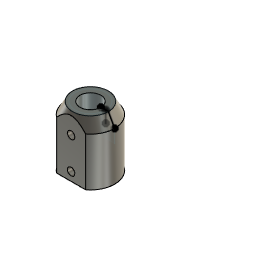
PuffingNozzle (Autodesk Fusion 360 design; units mm, degrees)
Autodesk Fusion 360 part; units mm, degrees
sketch "Sketch1" plane through (0, 0, 0) normal (0, 1, 0) x (1, 0, 0)
sketch "Sketch2" plane through (0, 0, 0) normal (0, 0, 1) x (1, 0, 0)
  circle A0 centre (-17.8237, 9.2304) radius 2.7432
  circle A1 centre (-17.8237, 9.2304) radius 6.35
  line L0 (-21.6337, 4.1504) -> (-14.0137, 4.1504)
  dimension "d3" = 5.4864
  dimension "d4" = 12.7
  dimension "d5" = 5.08
  constraint concentric A0 A1
  constraint coincident A1 L0.start
  constraint coincident A1 L0.end
  constraint horizontal L0
  measures "d3" diameter of A0
  measures "d4" diameter of A1
  measures "d5" distance of A0.centre L0
ref_plane "WorkPlane1" through (-17.8237, 9.2304, 2.9972) normal (0, 0, 1) x (1, 0, 0)
sketch "Sketch3" plane through (-17.8237, 9.2304, 2.9972) normal (0, 0, 1) x (1, 0, 0)
  circle A0 centre (0, 0) radius 4.0161
  constraint coincident A0.centre origin
extrude "Extrude1" add sketch "Sketch3" against normal up to surface (2.9972 mm away) makes body 1
extrude "Extrude2" cut sketch "Sketch2" along normal up to surface (2.9972 mm away) contours A0 bodies 1
extrude "Extrude3" add sketch "Sketch2" against normal blind 3.4544 bodies 1
sketch "Sketch4" plane through (0, 0, 0) normal (1, 0, 0) x (0, 1, 0)
ref_plane "WorkPlane2" through (0, 9.2202, 0) normal (0, 1, 0) x (0, 0, 1)
extrude "Extrude4" cut sketch "Sketch2" against normal blind 0.889 contours A1 L0 picked at (-18.8394, 3.9867) bodies 1
ref_plane "WorkPlane3" through (-17.8237, 9.2304, -0.4445) normal (0, -1, 0) x (-1, 0, 0)
extrude "Extrude5" add 1 faces at (-18.8394, 3.9867, -0.889) along direction (0, 0, 1) up to surface (0.889 mm away) on bodies 1 bodies 1
sketch "Sketch5" plane through (-17.8237, 9.2304, -0.4445) normal (0, -1, 0) x (1, 0, 0)
split "Split1" by plane through (-17.8237, 9.2304, -0.4445) normal (0, -1, 0) bodies 1 makes body 2 at (-11.5053, 8.5982, -2.3029)
sketch "Sketch6" plane through (-17.8237, 9.2304, -0.4445) normal (0, -1, 0) x (1, 0, 0)
sketch "Sketch7" plane through (0, 9.2304, 0) normal (0, -1, 0) x (1, 0, 0)
  line L0 (-11.4737, -3.4544) -> (-11.4737, 0)
  line L1 (-11.4737, 0) -> (-13.8076, 0)
  line L2 (-13.8076, 0) -> (-13.8076, 2.9972)
  line L3 (-13.8076, 2.9972) -> (-15.0805, 2.9972)
  line L4 (-15.0805, 2.9972) -> (-15.0805, -3.4544)
  line L5 (-15.0805, -3.4544) -> (-11.4737, -3.4544)
  line L6 (-13.8076, 0) -> (-13.8076, 2.9972)
  line L7 (-15.0805, 2.9972) -> (-13.1247, 2.9972)
  line L8 (-13.1247, 2.9972) -> (-11.4737, 0)
  dimension "d38" = 2.9972
  dimension "d39" = 1.9558
  constraint coincident L1.end L2.start
  constraint perpendicular L1 L6
  constraint coincident L3.end L4.start
  constraint perpendicular L2 L7
  constraint coincident L0.end L1.start
  measures "d38" distance of L1.end L2.end
  measures "d39" distance of L3.end L7.end
revolve "Revolve1" add sketch "Sketch7" angle 360 about axis through (-17.8237, 9.2304, 4.4958) along (0, 0, -1) contours L0 L1 L2 L3 L4 L5 L6 L7 bodies 1 2
extrude "Extrude6" cut sketch "Sketch2" against normal blind 6.35 contours A1 L0 picked at (-18.8394, 3.9867) bodies 1
extrude "Extrude7" add sketch "Sketch2" along normal blind 2.8194 separate body contours A1 L0 picked at (-18.8394, 3.9867) makes body 3
extrude "Extrude8" cut 1 faces at (-18.8394, 3.9867, 2.8194) along direction (0, 0, -1) blind 6.9088 on bodies 3 bodies 1 3
extrude "Extrude9" cut 1 faces at (-17.7554, 4.9319, -3.4544) along direction (0, 0, 1) blind 3.4544 on bodies 1 bodies 1
extrude "Extrude10" add sketch "Sketch2" against normal blind 18.6182 contours A1 L0 picked at (-17.7554, 4.9319) bodies 1 3
sketch "Sketch8" plane through (0, 4.1504, 0) normal (0, -1, 0) x (1, 0, 0)
  circle A0 centre (-17.8237, -10.4648) radius 0.9779
  circle A1 centre (-17.8237, -2.159) radius 0.9779
  line L0 (-14.0137, 0) -> (-21.6337, 0)
  dimension "d30" = 1.9558
  dimension "d32" = 1.9558
  dimension "d44" = 2.159
  dimension "d51" = 8.3058
  measures "d30" diameter of A0
  measures "d32" diameter of A1
  measures "d44" distance of A1.centre L0
  measures "d51" distance of A0.centre A1.centre
extrude "Extrude11" cut 1 faces at (-17.892, 4.9319, -18.6182) along direction (0, 0, 1) blind 1.6256 on bodies 1 bodies 1
surface "Revolve2" add revolved angle 360 about axis through (-17.8237, 9.2304, 4.4958) along (0, 0, -5.9944) profiles "Sketch7" section 1 contours L1 L2 L6 L7 L8 separate body makes body 4
sketch "Sketch9" plane through (0, 4.1504, 0) normal (0, -1, 0) x (1, 0, 0)
  line L0 (-21.59, 0) -> (-14.478, 0)
  line L1 (-14.478, 0) -> (-14.478, -12.6238)
  line L2 (-14.478, -12.6238) -> (-21.59, -12.6238)
  line L3 (-21.59, -12.6238) -> (-21.59, 0)
  line L4 (-14.478, -12.6238) -> (-21.59, -12.6238)
  line L5 (-21.59, -12.6238) -> (-21.59, -17.018)
  line L6 (-21.59, -17.018) -> (-14.478, -17.018)
  line L7 (-14.478, -17.018) -> (-14.478, -12.6238)
  dimension "d41" = 12.6238
  constraint horizontal L0
  constraint vertical L1
  constraint horizontal L2
  constraint vertical L3
  constraint horizontal L4
  constraint vertical L5
  constraint horizontal L6
  constraint vertical L7
  measures "d41" distance of L0.start L2.end
extrude "Extrude12" cut sketch "Sketch9" against normal blind 20.447 contours L2 L4 L5 L6 L7 bodies 1
extrude "Extrude13" cut 1 faces at (-21.59, 10.9454, -14.0801) along direction (1, 0, 0) blind 15.748 and the other way blind 7.5946 on bodies 1 bodies 1
extrude "Extrude14" cut 1 faces at (-14.4304, 14.5023, -16.9926) along direction (0, 0, 1) up to surface (4.3688 mm away) on bodies 1 bodies 1
extrude "Extrude15" add 1 faces at (-17.7554, 4.9319, -12.6238) along direction (0, 0, -1) blind 0.0762 on bodies 1 bodies 1
sketch "Sketch10" plane through (0, 0, 2.9972) normal (0, 0, 1) x (-1, 0, 0)
  circle A0 centre (17.8237, -9.2304) radius 4.699
  circle A1 centre (17.8237, -9.2304) radius 4.0161
stitch "SurfaceStitch1" surfaces 4 tolerance 0.1016 makes body 5
combine "Combine1" operation add target body 1 tool bodies 5
extrude "Extrude16" cut sketch "Sketch2" along normal blind 2.286 contours A1 L0 picked at (-18.8394, 3.9867) bodies 1
sketch "Sketch11" plane through (0, 0, -12.7) normal (0, 0, -1) x (1, 0, 0)
  circle A0 centre (-17.8237, -9.2304) radius 2.7432
  arc A1 (-21.6337, -4.1504) -> (-14.0137, -4.1504) centre (-17.8237, -9.2304) ccw
  line L0 (-14.0137, -4.1504) -> (-21.6337, -4.1504)
  circle A2 centre (-17.8237, -9.2304) radius 0.9906
  circle A3 centre (-17.8237, -9.2304) radius 3.9826
  dimension "d57" = 1.9812
  constraint concentric A0 A2
  constraint concentric A2 A3
  measures "d57" diameter of A2
extrude "Extrude17" add sketch "Sketch11" against normal blind 11.8872 separate body contours A0 makes body 6
extrude "Extrude18" cut sketch "Sketch8" against normal blind 34.2646 bodies 1
equation "d28 = -0.615 in - 0.118 in"
equation "d41 = 0.615 in - 0.118 in"
equation "d51 = 0.25 in + 0.077 in"
